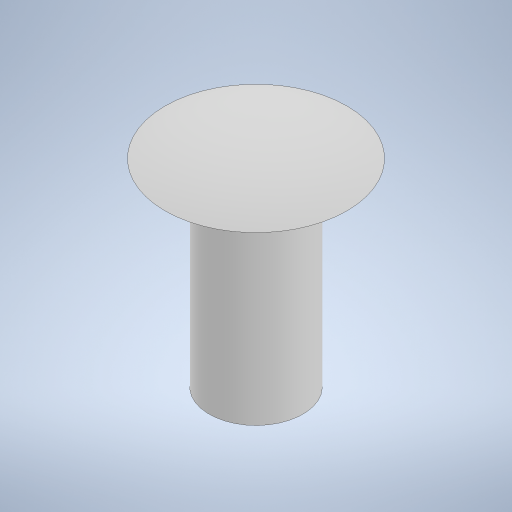
# Autodesk Inventor part: Rivet
Saved by Autodesk Inventor 2023 (Build 270158000, 158)
## iProperties
Created: 2022-11-03
Part Number: Rivet
Material: Generic
Document SubType Name: Modeling
Designer: Nebil
Density: 1 g/cm^3
Appearance: Default
Author: Nebil
Autodesk Inventor part; units mm, degrees
ref_plane "YZ Plane" through (0, 0, 0) normal (1, 0, 0) x (0, 1, 0)
ref_plane "XZ Plane" through (0, 0, 0) normal (0, 1, 0) x (-1, 0, 0)
ref_plane "XY Plane" through (0, 0, 0) normal (0, 0, 1) x (1, 0, 0)
sketch "Sketch1" plane through (0, 0, 0) normal (0, 1, 0) x (-1, 0, 0)
  circle A0 centre (0, 0) radius 2.5527
  dimension "d0" = 5.1054
  constraints: 1 centre point, 1 coincident
  measures "d0" diameter of A0
extrude "Extrusion1" add sketch "Sketch1" along normal blind 10.795
sketch "Sketch4" plane through (0, 0, 0) normal (1, 0, 0) x (0, 1, 0)
  line L0 (10.795, -2.5527) -> (10.795, 2.5527) projected
  line L1 (10.795, 0) -> (10.795, -4.953)
  line L2 (10.795, 0) -> (12.3825, 0)
  arc A0 (10.795, -4.953) -> (12.3825, 0) centre (3.998, -0.0436) ccw
  point P0 (0, 0)
  dimension "d5" = 4.953
  dimension "d6" = 1.5875
  constraints: 4 end point, 2 point on circle, 1 centre point, 1 collinear, 1 horizontal, 1 midpoint
  measures "d5" distance of L1.start L1.end
  measures "d6" distance of L1.start L2.end
revolve "Revolution1" add sketch "Sketch4" angle 360 about axis through (0, 10.795, 0) along (0, 1, 0)
body "Solid1"
